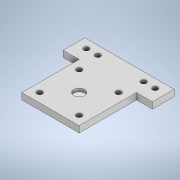
# Autodesk Inventor part: YAchseMotorteil
Saved by Autodesk Inventor 2021 (Build 250183000, 183)
## iProperties
Created: 2021-02-22
Part Number: YAchseMotorteil
Material: Generisch
Document SubType Name: Modeling
Designer: Kathrin H. Ulmer
Density: 1 g/cm^3
Appearance: Vorgabe
Author: Kathrin H. Ulmer
Autodesk Inventor part; units mm, degrees
ref_plane "YZ Plane" through (0, 0, 0) normal (1, 0, 0) x (0, 1, 0)
ref_plane "XZ Plane" through (0, 0, 0) normal (0, 1, 0) x (-1, 0, 0)
ref_plane "XY Plane" through (0, 0, 0) normal (0, 0, 1) x (1, 0, 0)
sketch "Skizze1" plane through (0, 0, 0) normal (0, 1, 0) x (-1, 0, 0)
  line L0 (4.2298, 8.039) -> (-65.7702, 8.039)
  line L1 (-65.7702, 8.039) -> (-65.7702, -8.961)
  line L2 (-65.7702, -8.961) -> (4.2298, -8.961)
  line L3 (4.2298, -8.961) -> (4.2298, 8.039)
  line L4 (-8.2702, 8.039) -> (-53.2702, 8.039)
  line L5 (-53.2702, 8.039) -> (-53.2702, 53.039)
  line L6 (-53.2702, 53.039) -> (-8.2702, 53.039)
  line L7 (-8.2702, 53.039) -> (-8.2702, 8.039)
  point P0 (0, 0)
  dimension "d0" = 70
  dimension "d1" = 17
  dimension "d2" = 45
  dimension "d3" = 45
  dimension "d4" = 12.5
  constraints: 16 end point, 4 parallel, 2 horizontal, 2 perpendicular, 1 point on line
  measures "d0" distance of L2.end L1.end
  measures "d1" distance between parallel lines of L0 L2
  measures "d2" distance of L5.end L6.end
  measures "d3" distance of L4.end L5.end
  measures "d4" distance between parallel lines of L3 L7
extrude "Extrusion1" add sketch "Skizze1" along normal blind 5
sketch "Skizze2" plane through (0, 5, 0) normal (0, 1, 0) x (1, 0, 0)
  point P0 (0, 0)
sketch "Skizze3" plane through (0, 5, 0) normal (0, 1, 0) x (1, 0, 0)
  circle A0 centre (0, 0) radius 2.1
  circle A1 centre (12.7702, 2.086) radius 2.1
  circle A2 centre (48.7702, 2.086) radius 2.1
  circle A3 centre (57.7702, 2.086) radius 2.1
  line L0 (65.7702, -8.039) -> (65.7702, 8.961) projected
  line L1 (65.7702, 8.961) -> (-4.2298, 8.961) projected
  line L2 (-4.2298, 8.961) -> (-4.2298, -8.039) projected
  dimension "d7" = 4.2
  dimension "d8" = 4.2
  dimension "d9" = 4.2
  dimension "d10" = 4.2
  dimension "d11" = 8
  dimension "d12" = 17
  dimension "d13" = 6.875
  dimension "d14" = 6.875
  dimension "d15" = 6.875
  dimension "d16" = 8.961
  dimension "d17" = 17
  constraints: 4 centre point, 1 coincident
  measures "d7" diameter of A0
  measures "d8" diameter of A1
  measures "d9" diameter of A2
  measures "d10" diameter of A3
  measures "d11" distance from line of L0 A3.centre
  measures "d12" distance from line of L0 A2.centre
  measures "d13" distance from line of L1 A2.centre
  measures "d14" distance from line of L1 A3.centre
  measures "d15" distance from line of L1 A1.centre
  measures "d16" distance from line of point (0, 0) L1
  measures "d17" distance from line of L2 A1.centre
sketch "Skizze4" plane through (0, 5, 0) normal (0, 1, 0) x (1, 0, 0)
  circle A0 centre (3.7702, 2.086) radius 2.1
  line L0 (65.7702, 8.961) -> (-4.2298, 8.961) projected
  line L1 (-4.2298, 8.961) -> (-4.2298, -8.039) projected
  point P0 (0, 0)
  dimension "d18" = 4.2
  dimension "d19" = 6.875
  dimension "d20" = 8
  constraints: 1 centre point
  measures "d18" diameter of A0
  measures "d19" distance from line of L0 A0.centre
  measures "d20" distance from line of L1 A0.centre
extrude "Extrusion2" cut sketch "Skizze4" against normal blind 20
extrude "Extrusion3" cut sketch "Skizze3" against normal blind 20 contours A1 | A2 | A3
sketch "Skizze5" plane through (0, 5, 0) normal (0, 1, 0) x (1, 0, 0)
  line L0 (9.6202, -51.689) -> (51.9202, -51.689)
  line L1 (51.9202, -51.689) -> (51.9202, -9.389)
  line L2 (51.9202, -9.389) -> (9.6202, -9.389)
  line L3 (9.6202, -9.389) -> (9.6202, -51.689)
  line L4 (8.2702, -8.039) -> (8.2702, -53.039) projected
  line L5 (8.2702, -53.039) -> (53.2702, -53.039) projected
  line L6 (15.2702, -46.039) -> (46.2702, -46.039)
  line L7 (46.2702, -46.039) -> (46.2702, -15.039)
  line L8 (46.2702, -15.039) -> (15.2702, -15.039)
  line L9 (15.2702, -15.039) -> (15.2702, -46.039)
  circle A0 centre (15.2702, -46.039) radius 2.125
  circle A1 centre (15.2702, -15.039) radius 2.125
  circle A2 centre (46.2702, -46.039) radius 2.125
  circle A3 centre (46.2702, -15.039) radius 2.125
  line L10 (15.2702, -46.039) -> (46.2702, -15.039)
  line L11 (46.2702, -46.039) -> (15.2702, -15.039)
  circle A4 centre (30.7702, -30.539) radius 4.25
  point P0 (0, 0)
  dimension "d25" = 42.3
  dimension "d26" = 42.3
  dimension "d27" = 1.35
  dimension "d28" = 1.35
  dimension "d29" = 31
  dimension "d30" = 31
  dimension "d31" = 5.65
  dimension "d32" = 5.65
  dimension "d33" = 4.25
  dimension "d34" = 4.25
  dimension "d35" = 4.25
  dimension "d36" = 4.25
  dimension "d37" = 8.5
  constraints: 20 end point, 5 centre point, 4 coincident, 4 parallel, 2 horizontal, 2 perpendicular, 1 midpoint
  measures "d25" distance of L2.end L1.end
  measures "d26" distance of L1.end L0.end
  measures "d27" distance between parallel lines of L4 L3
  measures "d28" distance between parallel lines of L5 L0
  measures "d29" distance of L8.end L7.end
  measures "d30" distance of L7.end L6.end
  measures "d31" distance between parallel lines of L7 L1
  measures "d32" distance between parallel lines of L2 L8
  measures "d33" diameter of A0
  measures "d34" diameter of A1
  measures "d35" diameter of A2
  measures "d36" diameter of A3
  measures "d37" diameter of A4
extrude "Extrusion4" cut sketch "Skizze5" against normal blind 20 contours L10 A0 L6 | L6 A0 L9 | L9 A0 L10 | A2 L11 L6 | L6 L7 A2 | A1 L8 L9 | L9 L11 A1 | A4 L11 L10 | L10 L11 A4 | L11 A2 L7 | L8 A1 L11 | L11 A4 L10 | L10 A4 L11 | A3 L7 L8 | L8 L10 A3 | A3 L10 L7
sketch "Skizze6" plane through (0, 0, 0) normal (0, -1, 0) x (1, 0, 0)
  circle A0 centre (46.2702, 46.039) radius 2.125 projected
  circle A1 centre (15.2702, 15.039) radius 2.125 projected
  line L0 (46.2702, 46.039) -> (15.2702, 46.039)
  line L1 (15.2702, 46.039) -> (15.2702, 15.039)
  line L2 (15.2702, 15.039) -> (46.2702, 15.039)
  line L3 (46.2702, 15.039) -> (46.2702, 46.039)
  line L4 (15.2702, 15.039) -> (46.2702, 46.039)
  line L5 (46.2702, 15.039) -> (15.2702, 46.039)
  circle A2 centre (30.7702, 30.539) radius 12
  point P0 (0, 0)
  dimension "d40" = 24
  constraints: 12 end point, 2 parallel, 2 perpendicular, 1 centre point, 1 horizontal, 1 midpoint
  measures "d40" diameter of A2
extrude "Extrusion5" cut sketch "Skizze6" against normal blind 2.5 contours A2 L5 L4 | L4 L5 A2 | L5 L4 A2 | A2 L4 L5
